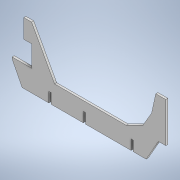
# Autodesk Inventor part: balkaRami
Saved by Autodesk Inventor 2020 (Build 240168000, 168)
## iProperties
Created: 2022-10-22
Part Number: balkaRami
Material: Типовые
Document SubType Name: Modeling
Designer: Inventor-2
Density: 1 g/cm^3
Appearance: По умолчанию
Author: Deep_
Обозначение: plaska
Разработал: Deep_
Стадия проекта: В работе
Дата создания: 02/12/2022
Autodesk Inventor part; units mm, degrees
ref_plane "YZ Plane" through (0, 0, 0) normal (1, 0, 0) x (0, 1, 0)
ref_plane "XZ Plane" through (0, 0, 0) normal (0, 1, 0) x (-1, 0, 0)
ref_plane "XY Plane" through (0, 0, 0) normal (0, 0, 1) x (1, 0, 0)
sketch "Видимый контур (ГОСТ)" plane through (0, 0, 0) normal (0, 0, 1) x (1, 0, 0)
  line L0 (177.4789, 341.3606) -> (207.4789, 341.3606)
  line L1 (177.4789, 411.3606) -> (177.4789, 341.3606)
  line L2 (206.442, 411.3606) -> (177.4789, 411.3606)
  line L3 (668.9949, 411.3606) -> (653.6245, 341.3606)
  line L4 (706.2543, 411.3606) -> (668.9949, 411.3606)
  line L5 (207.4789, 341.3606) -> (207.4789, 262.6394)
  line L6 (133.7457, 256.934) -> (171.2127, 182.6394)
  line L7 (133.7457, 262.6394) -> (133.7457, 256.934)
  line L8 (584.9543, 182.6394) -> (633.1308, 182.6394)
  line L9 (678.8529, 262.6394) -> (706.2543, 262.6394)
  line L10 (207.4789, 262.6394) -> (133.7457, 262.6394)
  line L11 (171.2127, 182.6394) -> (270.9543, 182.6394)
  line L12 (270.9543, 182.6394) -> (270.9543, 219.9127)
  line L13 (278.9543, 219.9127) -> (278.9543, 182.6394)
  line L14 (278.9543, 182.6394) -> (398.9543, 182.6394)
  line L15 (398.9543, 182.6394) -> (398.9543, 219.9127)
  line L16 (406.9543, 219.9127) -> (406.9543, 182.6394)
  line L17 (406.9543, 182.6394) -> (576.9543, 182.6394)
  line L18 (576.9543, 182.6394) -> (576.9543, 219.9127)
  line L19 (584.9543, 219.9127) -> (584.9543, 182.6394)
  line L20 (706.2543, 262.6394) -> (706.2543, 411.3606)
  line L21 (633.1308, 182.6394) -> (678.8529, 262.6394)
  line L22 (291.8603, 254.6406) -> (206.442, 411.3606)
  line L23 (558.5714, 254.6406) -> (291.8603, 254.6406)
  line L24 (621.3645, 286.3999) -> (558.5714, 254.6406)
  line L25 (653.6245, 341.3606) -> (621.3645, 286.3999)
  line L26 (270.9543, 219.9127) -> (278.9543, 219.9127)
  line L27 (398.9543, 219.9127) -> (406.9543, 219.9127)
  line L28 (576.9543, 219.9127) -> (584.9543, 219.9127)
  constraints: 58 end point
extrude "Выдавливание1" add sketch "Видимый контур (ГОСТ)" along normal blind 8
